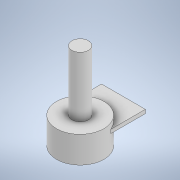
# Autodesk Inventor part: Potentiometer_Model
Saved by Autodesk Inventor 2021 (Build 250183000, 183)
## iProperties
Created: 2020-07-08
Part Number: Potentiometer_Model
Material: Generic
Document SubType Name: Modeling
Designer: ameli
Density: 1 g/cm^3
Appearance: Default
Author: ameli
Autodesk Inventor part; units mm, degrees
ref_plane "YZ Plane" through (0, 0, 0) normal (1, 0, 0) x (0, 1, 0)
ref_plane "XZ Plane" through (0, 0, 0) normal (0, 1, 0) x (-1, 0, 0)
ref_plane "XY Plane" through (0, 0, 0) normal (0, 0, 1) x (1, 0, 0)
sketch "Sketch1" plane through (0, 0, 0) normal (0, 1, 0) x (-1, 0, 0)
  circle A0 centre (0, 0) radius 8.25
  dimension "d0" = 16.5
  constraints: 1 centre point, 1 coincident
  measures "d0" diameter of A0
extrude "Extrusion1" add sketch "Sketch1" along normal blind 7.3
sketch "Sketch3" plane through (0, 7.3, 0) normal (0, 1, 0) x (1, 0, 0)
  line L0 (-7.65, 3) -> (7.65, 3)
  line L1 (7.65, 3) -> (7.65, 15.1)
  line L2 (7.65, 15.1) -> (-7.65, 15.1)
  line L3 (-7.65, 15.1) -> (-7.65, 3)
  point P0 (0, 0)
  dimension "d3" = 15.3
  dimension "d4" = 3
  dimension "d5" = 7.65
  dimension "d6" = 12.1
  constraints: 8 end point, 2 parallel, 1 horizontal, 1 perpendicular
  measures "d3" distance of L0.start L0.end
  measures "d4" distance from line of point (0, 0) L0
  measures "d5" distance from line of point (0, 0) L3
  measures "d6" distance of L2.end L0.start
extrude "Extrusion2" add sketch "Sketch3" against normal blind 1.3
sketch "Sketch4" plane through (0, 7.3, 0) normal (0, 1, 0) x (1, 0, 0)
  circle A0 centre (0, 0) radius 8.25
  dimension "d9" = 16.5
  constraints: 1 centre point, 1 coincident
  measures "d9" diameter of A0
extrude "Extrusion3" add sketch "Sketch4" along normal blind 2
sketch "Sketch5" plane through (0, 9.3, 0) normal (0, 1, 0) x (1, 0, 0)
  circle A0 centre (0, 0) radius 2.9
  dimension "d12" = 5.8
  constraints: 1 centre point, 1 coincident
  measures "d12" diameter of A0
extrude "Extrusion4" add sketch "Sketch5" along normal blind 21
body "Solid1"
